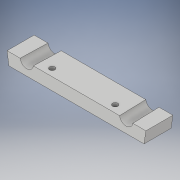
# Autodesk Inventor part: Bar_Mount_Bottom
Saved by Autodesk Inventor 2019 (Build 230136000, 136)
## iProperties
Created: 2019-08-14
Part Number: Bar_Mount_Bottom
Material: Generic
Document SubType Name: Modeling
Designer: steve
Density: 1 g/cm^3
Appearance: Default
Author: steve
Autodesk Inventor part; units mm, degrees
ref_plane "YZ Plane" through (0, 0, 0) normal (1, 0, 0) x (0, 1, 0)
ref_plane "XZ Plane" through (0, 0, 0) normal (0, 1, 0) x (-1, 0, 0)
sketch "Sketch1" plane through (0, 0, 0) normal (0, 0, 1) x (1, 0, 0)
  line L0 (75, -6.6976) -> (-75, -6.6976)
  line L1 (-75, -6.6976) -> (-77.0141, 6.8774)
  line L2 (-77.0141, 6.8774) -> (-61.6574, 6.8774)
  line L3 (77.0141, 6.8774) -> (75, -6.6976)
  line L4 (75, -6.6976) -> (-77.0141, 6.8774) construction
  line L5 (-75, -6.6976) -> (77.0141, 6.8774) construction
  line L6 (-77.1625, 7.8774) -> (77.8086, 7.8774) construction
  arc A0 (-46.9426, 6.8774) -> (-61.6574, 6.8774) centre (-54.3, 7.8774) ccw construction
  arc A1 (47.8105, 4.2695) -> (61.6574, 6.8774) centre (54.3, 7.8774) ccw
  line L7 (46.9426, 6.8774) -> (61.6574, 6.8774) construction
  line L8 (61.6574, 6.8774) -> (77.0141, 6.8774)
  arc A2 (46.9426, 6.8774) -> (47.8105, 4.2695) centre (54.3, 7.8774) ccw
  arc A3 (61.6574, 6.8774) -> (46.9426, 6.8774) centre (54.3, 7.8774) ccw construction
  line L9 (-61.6574, 6.8774) -> (-46.9426, 6.8774) construction
  line L10 (-46.9426, 6.8774) -> (46.9426, 6.8774)
  arc A4 (-47.8105, 4.2695) -> (-46.9426, 6.8774) centre (-54.3, 7.8774) ccw
  arc A5 (-61.3261, 5.4765) -> (-47.8105, 4.2695) centre (-54.3, 7.8774) ccw
  arc A6 (-61.6574, 6.8774) -> (-61.3261, 5.4765) centre (-54.3, 7.8774) ccw
  point P0 (0, 0)
  dimension "d0" = 1
  dimension "d1" = 14.85
  dimension "d2" = 54.3
  dimension "d3" = 108.6
  dimension "d5" = 150
  dimension "d6" = 22.7141
  dimension "d7" = 22.7141
  dimension "d8" = 14.575
  constraints: 22 end point, 15 point on circle, 8 point on line, 7 centre point, 6 horizontal, 5 parallel, 1 equal radius
  measures "d0" distance between parallel lines of L6 L2
  measures "d1" diameter of A0
  measures "d2" horizontal distance of point (0, 0) A0.centre
  measures "d3" distance of A1.centre A0.centre
  measures "d5" distance of L0.start L0.end
  measures "d6" horizontal distance of L1.end A0.centre
  measures "d7" horizontal distance of L3.start A1.centre
  measures "d8" distance from line of A0.centre L0
ref_plane "Work Plane1" through (0, 0, 30) normal (0, 0, 1) x (1, 0, 0)
sketch "Sketch2" plane through (0, 0, 30) normal (0, 0, 1) x (1, 0, 0)
  line L0 (75, -6.6976) -> (-75, -6.6976) projected
  line L1 (-75, -6.6976) -> (-77.0141, 6.8774) projected
  line L2 (77.0141, 6.8774) -> (75, -6.6976) projected
  line L3 (62.5574, 6.8774) -> (77.0141, 6.8774)
  line L4 (-47.8426, 6.8774) -> (47.8426, 6.8774)
  line L5 (-77.0141, 6.8774) -> (-62.5574, 6.8774)
  line L6 (-77.1625, 7.8774) -> (77.8086, 7.8774) construction
  arc A0 (-62.5574, 6.8774) -> (-47.8426, 6.8774) centre (-55.2, 7.8774) ccw
  arc A1 (47.8426, 6.8774) -> (62.5574, 6.8774) centre (55.2, 7.8774) ccw
  point P0 (0, 0)
  dimension "d10" = 7.425
  dimension "d11" = 110.4
  dimension "d12" = 55.2
  constraints: 6 end point, 4 point on circle, 2 centre point, 2 collinear, 2 point on line, 1 equal radius
  measures "d10" radius of A0
  measures "d11" distance of A1.centre A0.centre
  measures "d12" horizontal distance of A0.centre point (0, 0)
loft "Loft1" add profiles "Sketch1", "Sketch2"
sketch "Sketch8" plane through (-75, -6.6976, 0) normal (0, -1, 0) x (1, 0, 0)
  circle A0 centre (110, 22) radius 3
  circle A1 centre (40, 22) radius 3
  point P0 (75, 0)
  dimension "d31" = 35
  dimension "d32" = 35
  dimension "d33" = 22
  dimension "d34" = 22
  dimension "d35" = 6
  constraints: 2 centre point, 1 equal radius
  measures "d31" horizontal distance of point (75, 0) A0.centre
  measures "d32" horizontal distance of point (75, 0) A1.centre
  measures "d33" vertical distance of point (75, 0) A0.centre
  measures "d34" vertical distance of point (75, 0) A1.centre
  measures "d35" diameter of A0
extrude "Extrusion3" cut sketch "Sketch8" against normal through all
sketch "Sketch9" plane through (-75, -6.6976, 0) normal (0, -1, 0) x (1, 0, 0)
  circle A0 centre (110, 22) radius 3 projected
  circle A1 centre (40, 22) radius 3 projected
  line L0 (107.1132, 27) -> (112.8868, 27)
  line L1 (112.8868, 27) -> (115.7735, 22)
  line L2 (115.7735, 22) -> (112.8868, 17)
  line L3 (112.8868, 17) -> (107.1132, 17)
  line L4 (107.1132, 17) -> (104.2265, 22)
  line L5 (104.2265, 22) -> (107.1132, 27)
  line L6 (37.1132, 27) -> (42.8868, 27)
  line L7 (42.8868, 27) -> (45.7735, 22)
  line L8 (45.7735, 22) -> (42.8868, 17)
  line L9 (42.8868, 17) -> (37.1132, 17)
  line L10 (37.1132, 17) -> (34.2265, 22)
  line L11 (34.2265, 22) -> (37.1132, 27)
  point P0 (75, 0)
  dimension "d38" = 10
  constraints: 24 end point, 2 coincident, 2 horizontal, 1 collinear, 26 other
  measures "d38" distance between parallel lines of L0 L3
extrude "Extrusion4" cut sketch "Sketch9" against normal blind 5 and the other way blind 100
equation "\"d2\" = 0.5 * d3"
equation "\"d7\" = d6"
equation "\"d10\" = 0.5 * d1"
equation "\"d12\" = 0.5 * d11"
equation "\"d32\" = d31"
equation "\"d34\" = d33"
body "Solid1"
